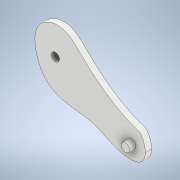
# Autodesk Inventor part: Component34
Saved by Autodesk Inventor 2022 (Build 260153000, 153)
## iProperties
Created: 2022-01-29
Part Number: Component34
Material: Generic
Document SubType Name: Modeling
Designer: Administrator
Density: 1 g/cm^3
Appearance: Default
Title: Component34
Author: Administrator
Autodesk Inventor part; units mm, degrees
ref_plane "YZ Plane" through (0, 0, 0) normal (1, 0, 0) x (0, 1, 0)
ref_plane "XZ Plane" through (0, 0, 0) normal (0, 1, 0) x (-1, 0, 0)
ref_plane "XY Plane" through (0, 0, 0) normal (0, 0, 1) x (1, 0, 0)
sketch "Sketch2" plane through (0, 0, 0) normal (0, 0, 1) x (1, 0, 0)
  circle A0 centre (-27.0693, 13.6896) radius 3.25
  circle A1 centre (33.5358, -15.7531) radius 3.25
  spline S0 degree 5 poles (44.2002, -16.3893) (44.2002, -15.3729) (44.0215, -13.3203) (43.2913, -10.297) (41.8291, -6.8845) (40.1428, -4.5044) (38.7042, -3.8955) (35.6627, -3.0769) (30.6292, -1.1867) (23.8745, 2.1071) (16.1954, 6.6344) (8.5229, 11.964) (1.665, 17.5427) (-4.071, 22.9013) (-8.8189, 27.681) (-12.9585, 31.6094) (-16.965, 34.4925) (-21.2416, 36.2007) (-25.9569, 36.6581) (-30.8853, 35.8303) (-35.569, 33.727) (-39.4809, 30.4046) (-42.1726, 25.9694) (-43.4646, 20.5779) (-43.389, 14.4574) (-42.0736, 7.922) (-39.6189, 1.4128) (-36.0391, -4.5234) (-31.0125, -9.0875) (-24.7806, -12.1023) (-17.8833, -13.79) (-10.9857, -14.6371) (-4.6627, -15.2295) (0.7673, -16.1083) (5.5095, -17.5972) (10.1628, -19.742) (15.3887, -22.3524) (21.5632, -24.9589) (28.6098, -26.9194) (35.3212, -27.1766) (40.5958, -25.3033) (43.1433, -22.2651) (44.0215, -19.419) (44.2002, -17.4058) (44.2002, -16.3893) knots 0 0 0 0 0 0 0.025 0.05 0.075 0.1 0.125 0.15 0.175 0.2 0.225 0.25 0.275 0.3 0.325 0.35 0.375 0.4 0.425 0.45 0.475 0.5 0.525 0.55 0.575 0.6 0.625 0.65 0.675 0.7 0.725 0.75 0.775 0.8 0.825 0.85 0.875 0.9 0.925 0.95 0.975 1 1 1 1 1 1 weights 1 1 1 1 1 1 1 1 1 1 1 1 1 1 1 1 1 1 1 1 1 1 1 1 1 1 1 1 1 1 1 1 1 1 1 1 1 1 1 1 1 1 1 1 1
  point P0 (0, 0)
  dimension "d4" = 6.5
  constraints: 2 centre point, 1 equal radius, 1 other
  measures "d4" diameter of A0
extrude "Extrusion1" add sketch "Sketch2" against normal blind 5 contours A1 | S0
extrude "Extrusion2" add sketch "Sketch2" along normal blind 5 contours A1
equation "\"d4\" = R"
equation "\"d0\" = thickness"
equation "\"d2\" = thickness"
equation "\"R\" = 6.5"
equation "\"thickness\" = 5"
equation "\"width\" = 6.5"
equation "\"R1\" = 9"
body "Solid1"
